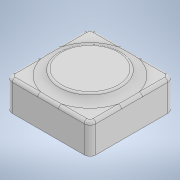
# Autodesk Inventor part: Small_Button
Saved by Autodesk Inventor 2021 (Build 250183000, 183)
## iProperties
Created: 2020-05-31
Part Number: Small_Button
Material: Generic
Document SubType Name: Modeling
Designer: ameli
Density: 1 g/cm^3
Appearance: Default
Author: ameli
Autodesk Inventor part; units mm, degrees
ref_plane "YZ Plane" through (0, 0, 0) normal (1, 0, 0) x (0, 1, 0)
ref_plane "XZ Plane" through (0, 0, 0) normal (0, 1, 0) x (-1, 0, 0)
ref_plane "XY Plane" through (0, 0, 0) normal (0, 0, 1) x (1, 0, 0)
sketch "Sketch5" plane through (0, 0, 0) normal (0, 1, 0) x (-1, 0, 0)
  line L0 (0, 0) -> (14, 0)
  line L1 (14, 0) -> (14, -14)
  line L2 (14, -14) -> (0, -14)
  line L3 (0, -14) -> (0, 0)
  dimension "d3" = 14
  dimension "d4" = 14
  constraints: 8 end point, 2 parallel, 1 horizontal, 1 perpendicular
  measures "d3" distance of L1.end L2.end
  measures "d4" distance of L0.end L1.end
extrude "Extrusion1" add sketch "Sketch5" along normal blind 5
sketch "Sketch6" plane through (0, 5, 0) normal (0, 1, 0) x (1, 0, 0)
  circle A0 centre (-7, 7) radius 5
  line L0 (0, 0) -> (0, 14) projected
  line L1 (0, 14) -> (-14, 14) projected
  dimension "d7" = 10
  dimension "d8" = 7
  dimension "d9" = 7
  constraints: 1 centre point
  measures "d7" diameter of A0
  measures "d8" distance from line of L0 A0.centre
  measures "d9" distance from line of L1 A0.centre
extrude "Extrusion2" add sketch "Sketch6" along normal blind 1
fillet "Fillet1" radius 2 1 edges at (-12, 5, -7)
fillet "Fillet2" radius 1 4 edges at (-14, 2.5, 0) (0, 2.5, 0) (-14, 2.5, -14) (0, 2.5, -14)
fillet "Fillet3" radius 0.5 9 edges at (-12, 6, -7) (-0.2929, 5, -13.7071) (-7, 5, -14) (-13.7071, 5, -13.7071) (-14, 5, -7) (-13.7071, 5, -0.2929) (-7, 5, 0) (-0.2929, 5, -0.2929) (0, 5, -7)
ref_plane "Work Plane2" through (-7, 0, -1) normal (1, 0, 0) x (0, 0, -1)
sketch "Sketch25" plane through (0, 0, 0) normal (0, -1, 0) x (1, 0, 0)
  line L0 (-4, -10) -> (-10, -10)
  line L1 (-10, -10) -> (-10, -4)
  line L2 (-10, -4) -> (-4, -4)
  line L3 (-4, -4) -> (-4, -10)
  line L4 (-1, -14) -> (-13, -14) projected
  line L5 (0, -1) -> (0, -13) projected
  point P0 (0, 0)
  dimension "d47" = 6
  dimension "d48" = 6
  dimension "d49" = 4
  dimension "d50" = 4
  constraints: 8 end point, 2 parallel, 1 horizontal, 1 perpendicular
  measures "d47" distance of L0.start L0.end
  measures "d48" distance of L0.end L1.end
  measures "d49" distance between parallel lines of L4 L0
  measures "d50" distance between parallel lines of L5 L3
extrude "Extrusion6" cut sketch "Sketch25" against normal blind 4.5
body "Solid1"
